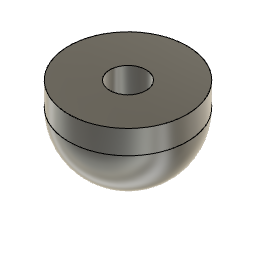
Halbkugel 1cm Durchmesser - Praktikanten Projekt v1 (Autodesk Fusion 360 design; units mm, degrees)
Autodesk Fusion 360 part; units mm, degrees
sketch "Skizze1" plane through (0, 0, 0) normal (0, 0, 1) x (1, 0, 0)
sketch "Skizze2" plane through (0, 0, 0) normal (0, 0, 1) x (1, 0, 0)
  circle A0 centre (0, 0) radius 5
  constraint coincident A0.centre origin
extrude "Extrusion1" add sketch "Skizze2" against normal blind 5
fillet "Abrundung1" radius 5 1 edges at (-4.6616, 1.8081, -5)
sketch "Skizze3" plane through (0, 0, 0) normal (0, 0, 1) x (-1, 0, 0)
  circle A0 centre (0, 0) radius 5
  circle A1 centre (0, 0) radius 1.525
  dimension "d5" = 3.05
  constraint concentric A0 A1
  measures "d5" diameter of A1
extrude "Extrusion2" add sketch "Skizze3" along normal blind 2
extrude "Extrusion3" cut 1 faces at (0.5137, -0.5901, 0) along direction (0, 0, -1) blind 4
